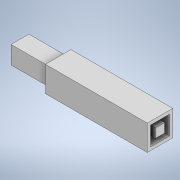
# Autodesk Inventor part: Center Piece
Saved by Autodesk Inventor 2022 (Build 260153000, 153)
## iProperties
Created: 2022-01-02
Part Number: Center Piece
Material: Generic
Document SubType Name: Modeling
Designer: josephinew
Density: 1 g/cm^3
Appearance: Default
Author: josephinew
Autodesk Inventor part; units mm, degrees
ref_plane "YZ Plane" through (0, 0, 0) normal (1, 0, 0) x (0, 1, 0)
ref_plane "XZ Plane" through (0, 0, 0) normal (0, 1, 0) x (-1, 0, 0)
ref_plane "XY Plane" through (0, 0, 0) normal (0, 0, 1) x (1, 0, 0)
sketch "Sketch1" plane through (0, 0, 0) normal (1, 0, 0) x (0, 1, 0)
  line L0 (0, 0) -> (25.4, 0)
  line L1 (25.4, 0) -> (25.4, -25.4)
  line L2 (25.4, -25.4) -> (0, -25.4)
  line L3 (0, -25.4) -> (0, 0)
  dimension "d0" = 25.4
  dimension "d1" = 25.4
  constraints: 8 end point, 2 parallel, 1 horizontal, 1 perpendicular
  measures "d0" distance of L1.end L2.end
  measures "d1" distance of L0.end L1.end
extrude "Extrusion1" add sketch "Sketch1" along normal blind 101.6
sketch "Sketch2" plane through (0, 0, 0) normal (-1, 0, 0) x (0, 0, 1)
  line L0 (-25.4, 0) -> (-25.4, 25.4) projected
  line L1 (-25.4, 0) -> (-21.59, 0)
  line L2 (-21.59, 3.81) -> (-17.78, 3.81)
  line L3 (-21.59, 7.62) -> (-21.59, 3.81)
  line L4 (-3.81, 21.59) -> (-7.62, 21.59)
  line L5 (-3.81, 17.78) -> (-3.81, 21.59)
  line L6 (-21.59, 3.81) -> (-3.81, 3.81)
  line L7 (-3.81, 3.81) -> (-3.81, 21.59)
  line L8 (-3.81, 21.59) -> (-21.59, 21.59)
  line L9 (-21.59, 21.59) -> (-21.59, 3.81)
  line L10 (-17.78, 7.62) -> (-7.62, 7.62)
  line L11 (-7.62, 7.62) -> (-7.62, 17.78)
  line L12 (-7.62, 17.78) -> (-17.78, 17.78)
  line L13 (-17.78, 17.78) -> (-17.78, 7.62)
  point P0 (0, 0)
  point P1 (0, 25.4)
  constraints: 26 end point, 5 horizontal, 4 parallel, 2 perpendicular
extrude "Extrusion2" add sketch "Sketch2" along normal blind 38.1
sketch "Sketch3" plane through (101.6, 0, 0) normal (1, 0, 0) x (0, 0, -1)
  line L0 (0, 25.4) -> (0, 0) projected
  line L1 (25.4, 25.4) -> (0, 25.4) projected
  line L2 (3.302, 3.81) -> (3.302, 3.302)
  line L3 (3.302, 3.302) -> (3.81, 3.302)
  line L4 (3.302, 3.302) -> (22.098, 3.302)
  line L5 (22.098, 3.302) -> (22.098, 22.098)
  line L6 (22.098, 22.098) -> (3.302, 22.098)
  line L7 (3.302, 22.098) -> (3.302, 3.302)
  line L8 (8.128, 8.128) -> (17.272, 8.128)
  line L9 (17.272, 8.128) -> (17.272, 17.272)
  line L10 (17.272, 17.272) -> (8.128, 17.272)
  line L11 (8.128, 17.272) -> (8.128, 8.128)
  dimension "d32" = 0.508
  dimension "d33" = 0.508
  constraints: 20 end point, 4 parallel, 2 horizontal, 2 perpendicular
  measures "d32" distance of L3.end L2.end
  measures "d33" distance of L2.end L2.start
extrude "Extrusion3" cut sketch "Sketch3" against normal blind 38.1
body "Solid1"
